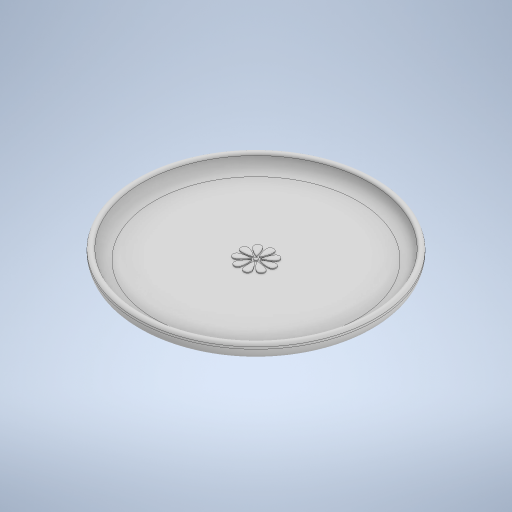
# Autodesk Inventor part: Plant Coaster V2
Saved by Autodesk Inventor 2024 (Build 280153000, 153)
## iProperties
Created: 2024-04-12
Part Number: Plant Coaster V2
Material: Generic
Document SubType Name: Modeling
Designer: haque
Density: 1 g/cm^3
Appearance: Default
Author: haque
Autodesk Inventor part; units mm, degrees
ref_plane "YZ Plane" through (0, 0, 0) normal (1, 0, 0) x (0, 1, 0)
ref_plane "XZ Plane" through (0, 0, 0) normal (0, 1, 0) x (-1, 0, 0)
ref_plane "XY Plane" through (0, 0, 0) normal (0, 0, 1) x (1, 0, 0)
sketch "Sketch1" plane through (0, 0, 0) normal (0, 1, 0) x (-1, 0, 0)
  circle A0 centre (0, 0) radius 67.5
  circle A1 centre (0, 0) radius 64.5
  dimension "d0" = 135
  dimension "d1" = 129
  constraints: 2 centre point, 2 coincident
  measures "d0" diameter of A0
  measures "d1" diameter of A1
extrude "Extrusion1" add sketch "Sketch1" along normal blind 10
extrude "Extrusion2" add sketch "Sketch1" along normal blind 3 contours A1
fillet "Fillet1" radius 7 2 edges at (67.5, 0, 0) (64.5, 3, 0)
fillet "Fillet2" radius 1.6 3 edges at (64.5, 10, 0) (64.5, 9.9995, 0) (67.5, 10, 0)
sketch "Sketch3" plane through (0, 3, 0) normal (0, 1, 0) x (1, 0, 0)
  circle A0 centre (0, 0) radius 10
  circle A1 centre (0, 0) radius 1
  line L0 (0, 0) -> (0, 10)
  circle A2 centre (0, 8) radius 2
  line L1 (2, 6) -> (-2, 6)
  line L2 (1, 3.5) -> (-1, 3.5)
  line L3 (0, 3.5) -> (0, -0.25)
  line L4 (0, 3.5) -> (0, 1.8333)
  line L5 (-2, 8) -> (-2, 6) construction
  line L6 (-2, 6) -> (-1, 3.5) construction
  line L7 (-1, 3.5) -> (0, 1.8333) construction
  spline S0 degree 3 poles (-2, 8) (-2, 6) (-1, 3.5) (0, 1.8333) knots 1 1 1 1 2 2 2 2
  line L8 (2, 8) -> (2, 6) construction
  line L9 (2, 6) -> (1, 3.5) construction
  line L10 (1, 3.5) -> (0, 1.8333) construction
  spline S1 degree 3 poles (2, 8) (2, 6) (1, 3.5) (0, 1.8333) knots 1 1 1 1 2 2 2 2
  dimension "d10" = 20
  dimension "d9" = 2
  dimension "d8" = 4
  constraints: 10 end point, 6 coincident, 3 point on line, 2 centre point, 2 point on circle, 2 tangent, 1 midpoint, 1 parallel, 1 perpendicular, 1 vertical, 1 vertical alignment, 8 other
  measures "d9" diameter of A1
  measures "d8" diameter of A2
extrude "Extrusion3" add sketch "Sketch3" along normal blind 0.5 contours A1 | A2 L0 | L0 A2 | L1 S1 L2 L0 | L1 S0 A2 | A2 S1 L1 | L0 L2 S0 L1 | L2 S1 L0 | L0 S0 L2
pattern_circular "Circular Pattern1" count 9 over 360 about axis through (0, -10, 0) along (0, 1, 0) of "Extrusion3"
body "Solid1"
